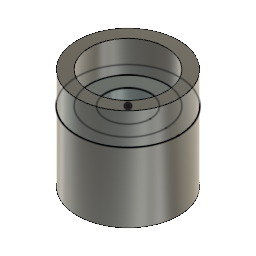
roller (Autodesk Fusion 360 design; units mm, degrees)
Autodesk Fusion 360 part; units mm, degrees
sketch "Sketch1" plane through (0, 0, 0) normal (0, 0, 1) x (1, 0, 0)
  circle A0 centre (0, 0) radius 1.75
  circle A1 centre (0, 0) radius 3
  circle A2 centre (0, 0) radius 4
  dimension "d1" = 3.5
  dimension "d2" = 6
  dimension "d3" = 8
  constraint coincident A0.centre A1.centre
  constraint concentric A0 A1
  constraint concentric A1 A2
  measures "d1" diameter of A0
  measures "d2" diameter of A1
  measures "d3" diameter of A2
extrude "Extrude1" add sketch "Sketch1" against normal blind 3 contours A1
extrude "Extrude2" add sketch "Sketch1" along normal blind 2.5 and the other way blind 5.5 contours A2
